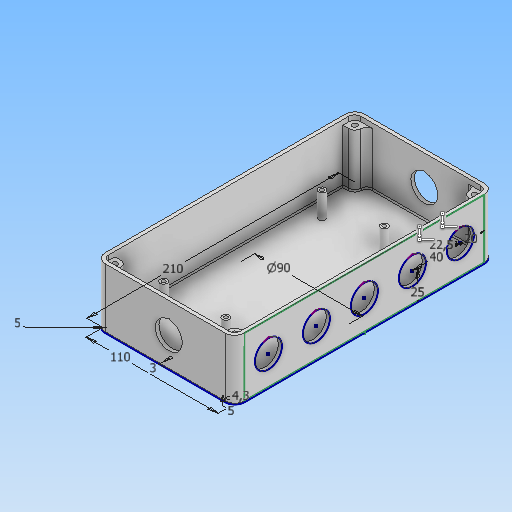
# Autodesk Inventor part: SchrackMulticlock_Box
Saved by Autodesk Inventor 2025.2 (Build 292293000, 293)
## iProperties
Created: 2024-12-26
Part Number: SchrackMulticlock_Box
Material: Všeobecné
Document SubType Name: Modeling
Designer: 42060
Density: 1 g/cm^3
Appearance: Výchozí
Author: 42060
Autodesk Inventor part; units mm, degrees
(part 1 of 2)
ref_plane "YZ Plane" through (0, 0, 0) normal (1, 0, 0) x (0, 1, 0)
ref_plane "XZ Plane" through (0, 0, 0) normal (0, 1, 0) x (-1, 0, 0)
ref_plane "XY Plane" through (0, 0, 0) normal (0, 0, 1) x (1, 0, 0)
sketch "PCB" plane through (0, 0, 0) normal (0, 1, 0) x (-1, 0, 0)
  line L0 (45, 45) -> (79, 45)
  line L1 (79, 45) -> (83.2426, 49.2426)
  line L2 (83.2426, 49.2426) -> (86.7426, 49.2426)
  line L3 (86.7426, 49.2426) -> (89.2426, 46.7426)
  line L4 (89.2426, 46.7426) -> (89.2426, 43.2426)
  line L5 (89.2426, 43.2426) -> (85, 39)
  line L6 (85, 39) -> (85, 0)
  circle A0 centre (85, 45) radius 1.6
  line L7 (85, 0) -> (45, 0)
  line L8 (45, 0) -> (45, 45)
  line L9 (45, -45) -> (79, -45)
  line L10 (79, -45) -> (83.2426, -49.2426)
  line L11 (83.2426, -49.2426) -> (86.7426, -49.2426)
  line L12 (86.7426, -49.2426) -> (89.2426, -46.7426)
  line L13 (89.2426, -46.7426) -> (89.2426, -43.2426)
  line L14 (89.2426, -43.2426) -> (85, -39)
  line L15 (85, -39) -> (85, 0)
  circle A1 centre (85, -45) radius 1.6
  line L16 (45, 45) -> (11, 45)
  line L17 (11, 45) -> (6.7574, 49.2426)
  line L18 (6.7574, 49.2426) -> (3.2574, 49.2426)
  line L19 (3.2574, 49.2426) -> (0.7574, 46.7426)
  line L20 (0.7574, 46.7426) -> (0.7574, 43.2426)
  line L21 (0.7574, 43.2426) -> (5, 39)
  line L22 (5, 39) -> (5, 0)
  circle A2 centre (5, 45) radius 1.6
  line L23 (45, -45) -> (11, -45)
  line L24 (11, -45) -> (6.7574, -49.2426)
  line L25 (6.7574, -49.2426) -> (3.2574, -49.2426)
  line L26 (3.2574, -49.2426) -> (0.7574, -46.7426)
  line L27 (0.7574, -46.7426) -> (0.7574, -43.2426)
  line L28 (0.7574, -43.2426) -> (5, -39)
  line L29 (5, -39) -> (5, 0)
  circle A3 centre (5, -45) radius 1.6
  line L30 (103.1723, 66.0113) -> (103.1723, -78.0847) construction
  line L31 (103.1723, -78.0847) -> (-10.5, -78.0847) construction
  line L32 (-10.5, -78.0847) -> (-10.5, 66.0113) construction
  line L33 (-10.5, 66.0113) -> (103.1723, 66.0113) construction
  line L34 (5, 40) -> (-75, 40)
  line L35 (-75, 40) -> (-75, -40)
  line L36 (-75, -40) -> (5, -40)
  line L37 (5, -40) -> (5, 40)
  line L38 (5, 40) -> (-75, -40) construction
  line L39 (-75, 40) -> (5, -40) construction
  circle A4 centre (-66, 31) radius 2
  line L40 (5, 0) -> (-75, 0)
  line L41 (-35, -40) -> (-35, 40)
  circle A5 centre (-66, -31) radius 2
  circle A6 centre (-4, 31) radius 2
  circle A7 centre (-4, -31) radius 2
  line L42 (-67.5, -40) -> (-67.5, 40) construction
  line L43 (-45, 55) -> (-90, 55)
  line L44 (-90, 55) -> (-90, 25)
  line L45 (-90, 25) -> (-45, 25)
  line L46 (-45, 25) -> (-45, 55)
  line L47 (-45, 55) -> (-90, 25) construction
  line L48 (-90, 55) -> (-45, 25) construction
  line L49 (-45, -15) -> (-45, 15)
  line L50 (-90, -15) -> (-45, -15)
  line L51 (-90, 15) -> (-90, -15)
  line L52 (-45, 15) -> (-90, 15)
  line L53 (-45, -55) -> (-45, -25)
  line L54 (-90, -55) -> (-45, -55)
  line L55 (-90, -25) -> (-90, -55)
  line L56 (-45, -25) -> (-90, -25)
  line L57 (76, 60.25) -> (14, 60.25)
  line L58 (14, 60.25) -> (14, 49.75)
  line L59 (14, 49.75) -> (76, 49.75)
  line L60 (76, 49.75) -> (76, 60.25)
  line L61 (76, 60.25) -> (14, 49.75) construction
  line L62 (14, 60.25) -> (76, 49.75) construction
  line L63 (-13.5, 26.75) -> (-56.5, 26.75)
  line L64 (-56.5, 26.75) -> (-56.5, -26.75)
  line L65 (-56.5, -26.75) -> (-13.5, -26.75)
  line L66 (-13.5, -26.75) -> (-13.5, 26.75)
  line L67 (-13.5, 26.75) -> (-56.5, -26.75) construction
  line L68 (-56.5, 26.75) -> (-13.5, -26.75) construction
  line L69 (-9, 26.75) -> (-61, 26.75)
  line L70 (-61, 26.75) -> (-61, -26.75)
  line L71 (-61, -26.75) -> (-9, -26.75)
  line L72 (-9, -26.75) -> (-9, 26.75)
  line L73 (-9, 26.75) -> (-61, -26.75) construction
  line L74 (-61, 26.75) -> (-9, -26.75) construction
  point P0 (0, 0)
  point P1 (0, 0)
  point P2 (-35, 0)
  point P3 (-67.5, 0)
  point P4 (45, 55)
  dimension "d2" = 6
  dimension "d3" = 39
  dimension "d4" = 34
  dimension "d5" = 40
  dimension "d6" = 45
  dimension "d7" = 3.5
  dimension "d8" = 3.2
  dimension "d11" = 45
  dimension "d65" = 80
  dimension "d66" = 80
  dimension "d68" = 80
  dimension "d69" = 4
  dimension "d70" = 31
  dimension "d83" = 55.5
  dimension "d87" = 144.096
  dimension "d91" = 66.0113
  dimension "d105" = 30
  dimension "d106" = 45
  dimension "d107" = 40
  dimension "d110" = 40
  dimension "d116" = 135
  dimension "d117" = 62
  dimension "d118" = 10.5
  dimension "d120" = 55
  dimension "d162" = 43
  dimension "d163" = 53.5
  dimension "d164" = 52
  constraints: 142 end point, 26 symmetric about line, 15 midpoint, 12 parallel, 9 horizontal, 9 perpendicular, 8 centre point, 5 horizontal alignment, 3 equal length, 3 vertical alignment, 2 vertical, 1 coincident, 1 point on line, 26 other
  measures "d2" distance of L4.end L5.end
  measures "d3" distance of L5.end L6.end
  measures "d4" distance of L0.start L0.end
  measures "d5" distance from line of L7.end L6
  measures "d6" distance from line of L7.end L0
  measures "d7" distance of L3.end L4.end
  measures "d8" diameter of A0
  measures "d11" distance of point (0, 0) L7.end
  measures "d65" distance of L35.end L36.end
  measures "d66" distance of L34.end L35.end
  measures "d68" distance of point (-35, 0) L7.end
  measures "d69" diameter of A4
  measures "d70" vertical distance of L40.end A4.centre
  measures "d83" distance from line of L7.end L32
  measures "d87" distance between parallel lines of L31 L33
  measures "d91" distance from line of L33 L7.end
  measures "d105" distance of L45.end L43.start
  measures "d106" distance of L44.end L45.end
  measures "d107" distance of L42.end point (-67.5, 0)
  measures "d110" distance of L45.end L49.start
  measures "d116" distance from line of L7.end L51
  measures "d117" distance of L58.end L59.end
  measures "d118" distance of L57.end L58.end
  measures "d120" distance of L7.end point (45, 55)
  measures "d162" distance of L63.start L63.end
  measures "d163" distance of L65.end L63.start
  measures "d164" distance of L70.end L71.end
sketch "Náčrt2" plane through (0, 0, 0) normal (0, 1, 0) x (-1, 0, 0)
  line L0 (50, 105) -> (-40, 105)
  line L1 (-55, 90) -> (-55, -100)
  line L2 (-50, -105) -> (50, -105)
  line L3 (55, -100) -> (55, 100)
  line L4 (55, 105) -> (-55, -105) construction
  line L5 (-55, 105) -> (55, -105) construction
  arc A0 (55, 100) -> (50, 105) centre (50, 100) ccw
  arc A1 (50, -105) -> (55, -100) centre (50, -100) ccw
  arc A2 (-55, -100) -> (-50, -105) centre (-50, -100) ccw
  arc A3 (-50, 105) -> (-55, 100) centre (-50, 100) ccw
  line L6 (-50, 108) -> (50, 108)
  arc A4 (58, 100) -> (50, 108) centre (50, 100) ccw
  line L7 (58, 100) -> (58, -100)
  arc A5 (50, -108) -> (58, -100) centre (50, -100) ccw
  line L8 (50, -108) -> (-50, -108)
  arc A6 (-58, -100) -> (-50, -108) centre (-50, -100) ccw
  line L9 (-58, -100) -> (-58, 100)
  arc A7 (-50, 108) -> (-58, 100) centre (-50, 100) ccw
  circle A8 centre (-50, 100) radius 5
  line L10 (-45, 100) -> (-45, 100)
  line L11 (-50, 95) -> (-50, 95)
  arc A9 (-40, 105) -> (-45, 100) centre (-40, 100) ccw
  arc A10 (-50, 95) -> (-55, 90) centre (-50, 90) ccw
  line L12 (-40, 105) -> (-50, 105)
  line L13 (-55, 90) -> (-55, 100)
  circle A11 centre (-50, 100) radius 2.15
  line L14 (55, 0) -> (-55, 0)
  line L15 (0, 105) -> (0, -105)
  circle A12 centre (-50, -100) radius 5
  arc A13 (-45, -100) -> (-40, -105) centre (-40, -100) ccw
  arc A14 (-55, -90) -> (-50, -95) centre (-50, -90) ccw
  circle A15 centre (-50, -100) radius 2.15
  circle A16 centre (50, 100) radius 5
  line L16 (45, 100) -> (45, 100)
  line L17 (50, 95) -> (50, 95)
  arc A17 (45, 100) -> (40, 105) centre (40, 100) ccw
  arc A18 (55, 90) -> (50, 95) centre (50, 90) ccw
  circle A19 centre (50, 100) radius 2.15
  arc A20 (50, -95) -> (55, -90) centre (50, -90) ccw
  circle A21 centre (50, -100) radius 2.15
  arc A22 (40, -105) -> (45, -100) centre (40, -100) ccw
  circle A23 centre (50, -100) radius 5
  line L18 (-50, 95) -> (-55, 95)
  line L19 (-50, -95) -> (-55, -95)
  line L20 (50, 95) -> (55, 95)
  line L21 (50, -95) -> (55, -95)
  point P0 (0, 0)
  point P1 (-45, 100)
  point P2 (-55, 100)
  point P3 (-45, -100)
  point P4 (-50, -95)
  point P5 (50, -100)
  point P6 (45, -100)
  point P7 (50, -95)
  point P8 (-40, -105)
  point P9 (-45, -100)
  point P10 (-50, -95)
  point P11 (50, -95)
  point P12 (40, -105)
  point P13 (45, 100)
  point P14 (40, 105)
  point P15 (55, 95)
  point P16 (50, -95)
  point P17 (-50, -95)
  point P18 (45, 0)
  point P19 (0, 0)
  dimension "d9" = 210
  dimension "d10" = 110
  dimension "d12" = 5
  dimension "d124" = 3
  dimension "d136" = 5
  dimension "d137" = 4.3
  dimension "d525" = 90
  constraints: 44 end point, 41 point on circle, 40 symmetric about line, 24 centre point, 16 tangent, 13 point on line, 8 coincident, 6 midpoint, 5 equal radius, 4 parallel, 4 perpendicular, 3 horizontal, 2 vertical, 1 horizontal alignment, 19 other
  measures "d9" distance of L5.end L4.start
  measures "d10" distance of L4.start L5.start
  measures "d12" radius of A0
  measures "d124" distance between parallel lines of L0 L6
  measures "d136" radius of A9
  measures "d137" diameter of A11
  measures "d525" diameter of point (45, 0) point (0, 0)
extrude "Vysunutí1" add sketch "Náčrt2" along normal blind 2 contours A16 A17 L0 | A0 A16 | A17 A16 A18 L3 L14 L15 L0 | L3 L20 A16 | L15 L14 L1 A10 A8 A9 L0 | L3 A18 L20 | A9 A8 L12 | L15 L2 A13 A12 A14 L1 L14 | L14 L3 A20 A23 A22 L2 L15 | A8 A3 | L18 L13 A8 | A10 L13 L18 | L3 L21 A20 | A14 L19 L1 | L2 A12 A13 | A22 A23 L2 | L3 A23 L21 | A23 A1 | L19 A12 L1 | A12 A2 | L6 A4 L7 A5 L8 A6 L9 A7 | A11 | A15 | A19 | A21
extrude "Vysunutí2" add sketch "Náčrt2" along normal blind 50 contours L6 A4 L7 A5 L8 A6 L9 A7
extrude "Vysunutí4" add sketch "Náčrt2" along normal blind 46 contours A16 A17 L0 | A0 A16 | L3 L20 A16 | A9 A8 L12 | A8 A3 | L18 L13 A8 | L2 A12 A13 | A22 A23 L2 | L3 A23 L21 | A23 A1 | L19 A12 L1 | A12 A2
chamfer "Zkosení1" distance 1 angle 45 8 edges at (58, 0, 0) (55.6569, 0, -105.6569) (0, 0, -108) (-55.6569, 0, -105.6569) (-58, 0, 0) (-55.6569, 0, 105.6569) (0, 0, 108) (55.6569, 0, 105.6569)
chamfer "Zkosení2" distance 1 angle 45 16 edges at (-46.4645, 2, 96.4645) (-43.5355, 2, 103.5355) (0, 2, 105) (43.5355, 2, 103.5355) (46.4645, 2, 96.4645) (52.5, 2, 95) (-52.5, 2, 95) (-55, 2, 0) (0, 2, -105) (-43.5355, 2, -103.5355) (-46.4645, 2, -96.4645) (-52.5, 2, -95) (43.5355, 2, -103.5355) (46.4645, 2, -96.4645) (52.5, 2, -95) (55, 2, 0)
ref_plane "Pracovní rovina1" through (0, 36, 0) normal (0, 1, 0) x (1, 0, 0)
sketch "Náčrt6" plane through (58, 50, 100) normal (1, 0, 0) x (0, 0, -1)
  circle A0 centre (180, -25) radius 11.25
  line L0 (176.0852, -14.4531) -> (180, -13)
  line L1 (180, -13) -> (183.9148, -14.4531)
  line L2 (0, -50) -> (200, -50) projected
  line L3 (200, -49) -> (200, 0) projected
  line L4 (200, -49) -> (0, -49) projected
  line L5 (200, -49) -> (200, 0) projected
  line L6 (0, 0) -> (200, 0) projected
  line L7 (0, -49) -> (0, 0) projected
  circle A1 centre (140, -25) radius 11.25
  line L8 (136.0852, -14.4531) -> (140, -13)
  line L9 (140, -13) -> (143.9148, -14.4531)
  circle A2 centre (100, -25) radius 11.25
  line L10 (96.0852, -14.4531) -> (100, -13)
  line L11 (100, -13) -> (103.9148, -14.4531)
  circle A3 centre (60, -25) radius 11.25
  line L12 (56.0852, -14.4531) -> (60, -13)
  line L13 (60, -13) -> (63.9148, -14.4531)
  circle A4 centre (20, -25) radius 11.25
  line L14 (16.0852, -14.4531) -> (20, -13)
  line L15 (20, -13) -> (23.9148, -14.4531)
  point P0 (100, -50)
  point P1 (182.4515, -14.0204)
  dimension "d609" = 22.5
  dimension "d610" = 25
  dimension "d611" = 20
  dimension "d614" = 40
  constraints: 20 end point, 10 point on circle, 5 centre point, 2 tangent, 1 horizontal, 28 other
  measures "d609" diameter of A0
  measures "d610" distance from line of L2 A0.centre
  measures "d611" distance from line of L3 A0.centre
  measures "d614" distance of A0.centre A1.centre
extrude "Vysunutí8" cut sketch "Náčrt6" against normal up to surface (3 mm away) contours A0 | A0 L0 L1 | A1 | A1 L8 L9 | A2 | A2 L10 L11 | A3 | A3 L12 L13 | A4 | A4 L14 L15
sketch "Sketch16" plane through (-58, 50, -100) normal (-1, 0, 0) x (0, 0, 1)
  line L0 (83.6122, -35.7493) -> (81.9759, -35.7493)
  line L1 (81.9759, -35.7493) -> (81.7423, -35.786)
  line L2 (81.7423, -35.786) -> (81.5927, -35.8771)
  line L3 (81.5927, -35.8771) -> (81.4287, -36.1113)
  line L4 (81.4287, -36.1113) -> (81.2378, -36.3119)
  line L5 (81.2378, -36.3119) -> (81.0126, -36.3763)
  line L6 (81.0126, -36.3763) -> (80.8497, -36.3769)
  line L7 (80.8497, -36.3769) -> (80.6856, -36.3485)
  line L8 (80.6856, -36.3485) -> (80.6027, -36.2609)
  line L9 (80.6027, -36.2609) -> (80.6707, -35.9053)
  line L10 (80.6707, -35.9053) -> (81.9875, -33.1293)
  line L11 (81.9875, -33.1293) -> (82.2034, -32.8403)
  line L12 (82.2034, -32.8403) -> (82.5118, -32.7443)
  line L13 (82.5118, -32.7443) -> (82.8391, -32.7481)
  line L14 (82.8391, -32.7481) -> (83.0353, -32.858)
  line L15 (83.0353, -32.858) -> (83.0612, -33.0921)
  line L16 (83.0612, -33.0921) -> (83.0433, -33.383)
  line L17 (83.0433, -33.383) -> (83.12, -33.4728)
  line L18 (83.12, -33.4728) -> (83.2556, -33.506)
  line L19 (83.2556, -33.506) -> (84.7242, -33.506)
  line L20 (84.7242, -33.506) -> (84.9963, -33.4315)
  line L21 (84.9963, -33.4315) -> (85.2006, -33.235)
  line L22 (85.2006, -33.235) -> (85.3303, -32.9572)
  line L23 (85.3303, -32.9572) -> (85.3787, -32.6387)
  line L24 (85.3787, -32.6387) -> (85.3391, -32.3203)
  line L25 (85.3391, -32.3203) -> (85.2049, -32.0425)
  line L26 (85.2049, -32.0425) -> (84.9692, -31.846)
  line L27 (84.9692, -31.846) -> (84.6255, -31.7714)
  line L28 (84.6255, -31.7714) -> (81.2636, -31.7714)
  line L29 (81.2636, -31.7714) -> (80.806, -31.8484)
  line L30 (80.806, -31.8484) -> (80.4005, -32.0677)
  line L31 (80.4005, -32.0677) -> (80.0566, -32.4122)
  line L32 (80.0566, -32.4122) -> (79.7838, -32.8649)
  line L33 (79.7838, -32.8649) -> (78.2065, -36.2017)
  line L34 (78.2065, -36.2017) -> (78.0796, -36.6902)
  line L35 (78.0796, -36.6902) -> (78.1692, -37.0583)
  line L36 (78.1692, -37.0583) -> (78.4033, -37.2907)
  line L37 (78.4033, -37.2907) -> (78.7097, -37.3716)
  line L38 (78.7097, -37.3716) -> (82.3161, -37.3716)
  line L39 (82.3161, -37.3716) -> (82.7872, -37.3019)
  line L40 (82.7872, -37.3019) -> (83.1788, -37.1181)
  line L41 (83.1788, -37.1181) -> (83.4864, -36.8583)
  line L42 (83.4864, -36.8583) -> (83.7057, -36.5605)
  line L43 (83.7057, -36.5605) -> (83.8322, -36.2626)
  line L44 (83.8322, -36.2626) -> (83.8618, -36.0028)
  line L45 (83.8618, -36.0028) -> (83.7899, -35.819)
  line L46 (83.7899, -35.819) -> (83.6122, -35.7493)
  line L47 (72.2106, -32.761) -> (72.4074, -32.7104)
  line L48 (72.4074, -32.7104) -> (72.5473, -32.5627)
  line L49 (72.5473, -32.5627) -> (72.5797, -32.4966)
  line L50 (72.5797, -32.4966) -> (72.6457, -32.3535)
  line L51 (72.6457, -32.3535) -> (72.6482, -32.349)
  line L52 (72.6482, -32.349) -> (72.7793, -32.0641)
  line L53 (72.7793, -32.0641) -> (72.7841, -31.8728)
  line L54 (72.7841, -31.8728) -> (72.7229, -31.8003)
  line L55 (72.7229, -31.8003) -> (72.609, -31.7714)
  line L56 (72.609, -31.7714) -> (70.745, -31.7657)
  line L57 (70.745, -31.7657) -> (70.7334, -31.7689)
  line L58 (70.7334, -31.7689) -> (67.6082, -31.7689)
  line L59 (67.6082, -31.7689) -> (66.5311, -31.7657)
  line L60 (66.5311, -31.7657) -> (66.4384, -31.7817)
  line L61 (66.4384, -31.7817) -> (66.3006, -31.8437)
  line L62 (66.3006, -31.8437) -> (66.1974, -31.9653)
  line L63 (66.1974, -31.9653) -> (66.1651, -32.0223)
  line L64 (66.1651, -32.0223) -> (66.0672, -32.2303)
  line L65 (66.0672, -32.2303) -> (66.0728, -32.2303)
  line L66 (66.0728, -32.2303) -> (65.9641, -32.4671)
  line L67 (65.9641, -32.4671) -> (65.9591, -32.6573)
  line L68 (65.9591, -32.6573) -> (66.0197, -32.73)
  line L69 (66.0197, -32.73) -> (66.1332, -32.759)
  line L70 (66.1332, -32.759) -> (66.5122, -32.7603)
  line L71 (66.5122, -32.7603) -> (66.5122, -32.761)
  line L72 (66.5122, -32.761) -> (67.4629, -32.761)
  line L73 (67.4629, -32.761) -> (67.9984, -32.7635)
  line L74 (67.9984, -32.7635) -> (67.9997, -32.761)
  line L75 (67.9997, -32.761) -> (68.0321, -32.761)
  line L76 (68.0321, -32.761) -> (66.0465, -37.0661)
  line L77 (66.0465, -37.0661) -> (66.0469, -37.2892)
  line L78 (66.0469, -37.2892) -> (66.2073, -37.3915)
  line L79 (66.2073, -37.3915) -> (66.4833, -37.3915)
  line L80 (66.4833, -37.3915) -> (67.8656, -37.3915)
  line L81 (67.8656, -37.3915) -> (67.9721, -37.3895)
  line L82 (67.9721, -37.3895) -> (68.1683, -37.3379)
  line L83 (68.1683, -37.3379) -> (68.3102, -37.19)
  line L84 (68.3102, -37.19) -> (68.5042, -36.7838)
  line L85 (68.5042, -36.7838) -> (68.5046, -36.7838)
  line L86 (68.5046, -36.7838) -> (68.5637, -36.6586)
  line L87 (68.5637, -36.6586) -> (68.5663, -36.6529)
  line L88 (68.5663, -36.6529) -> (68.8155, -36.1164)
  line L89 (68.8155, -36.1164) -> (68.856, -36.0285)
  line L90 (68.856, -36.0285) -> (68.9104, -35.9123)
  line L91 (68.9104, -35.9123) -> (69.9435, -33.6927)
  line L92 (69.9435, -33.6927) -> (70.3078, -32.9111)
  line L93 (70.3078, -32.9111) -> (70.398, -32.8193)
  line L94 (70.398, -32.8193) -> (70.5648, -32.7635)
  line L95 (70.5648, -32.7635) -> (70.8183, -32.7635)
  line L96 (70.8183, -32.7635) -> (70.8183, -32.761)
  line L97 (70.8183, -32.761) -> (71.9394, -32.761)
  line L98 (71.9394, -32.761) -> (72.2106, -32.761)
  line L99 (77.0928, -36.3955) -> (75.2413, -36.3955)
  line L100 (75.2413, -36.3955) -> (73.931, -36.3955)
  line L101 (73.931, -36.3955) -> (73.8331, -36.3352)
  line L102 (73.8331, -36.3352) -> (73.8323, -36.1979)
  line L103 (73.8323, -36.1979) -> (73.8693, -36.1164)
  line L104 (73.8693, -36.1164) -> (74.279, -35.2373)
  line L105 (74.279, -35.2373) -> (74.3685, -35.1443)
  line L106 (74.3685, -35.1443) -> (74.5372, -35.0884)
  line L107 (74.5372, -35.0884) -> (75.165, -35.0865)
  line L108 (75.165, -35.0865) -> (76.1951, -35.0865)
  line L109 (76.1951, -35.0865) -> (76.4663, -35.0865)
  line L110 (76.4663, -35.0865) -> (76.6641, -35.0349)
  line L111 (76.6641, -35.0349) -> (76.8056, -34.8875)
  line L112 (76.8056, -34.8875) -> (76.8341, -34.8214)
  line L113 (76.8341, -34.8214) -> (76.9022, -34.679)
  line L114 (76.9022, -34.679) -> (76.9048, -34.6726)
  line L115 (76.9048, -34.6726) -> (77.0773, -34.3228)
  line L116 (77.0773, -34.3228) -> (77.0823, -34.1311)
  line L117 (77.0823, -34.1311) -> (77.0216, -34.0581)
  line L118 (77.0216, -34.0581) -> (76.9091, -34.029)
  line L119 (76.9091, -34.029) -> (76.6871, -34.029)
  line L120 (76.6871, -34.029) -> (76.6897, -34.0264)
  line L121 (76.6897, -34.0264) -> (75.0378, -34.0264)
  line L122 (75.0378, -34.0264) -> (74.9399, -33.966)
  line L123 (74.9399, -33.966) -> (74.9387, -33.8281)
  line L124 (74.9387, -33.8281) -> (75.0469, -33.5913)
  line L125 (75.0469, -33.5913) -> (75.0413, -33.5939)
  line L126 (75.0413, -33.5939) -> (75.3621, -32.9124)
  line L127 (75.3621, -32.9124) -> (75.4507, -32.8201)
  line L128 (75.4507, -32.8201) -> (75.6173, -32.7648)
  line L129 (75.6173, -32.7648) -> (75.8696, -32.7635)
  line L130 (75.8696, -32.7635) -> (75.8696, -32.761)
  line L131 (75.8696, -32.761) -> (76.4163, -32.761)
  line L132 (76.4163, -32.761) -> (76.4529, -32.761)
  line L133 (76.4529, -32.761) -> (78.5752, -32.761)
  line L134 (78.5752, -32.761) -> (78.849, -32.761)
  line L135 (78.849, -32.761) -> (79.0453, -32.7104)
  line L136 (79.0453, -32.7104) -> (79.1853, -32.5627)
  line L137 (79.1853, -32.5627) -> (79.2159, -32.4966)
  line L138 (79.2159, -32.4966) -> (79.2823, -32.3535)
  line L139 (79.2823, -32.3535) -> (79.2849, -32.349)
  line L140 (79.2849, -32.349) -> (79.4164, -32.0641)
  line L141 (79.4164, -32.0641) -> (79.4213, -31.8728)
  line L142 (79.4213, -31.8728) -> (79.3604, -31.8003)
  line L143 (79.3604, -31.8003) -> (79.247, -31.7714)
  line L144 (79.247, -31.7714) -> (77.3821, -31.7657)
  line L145 (77.3821, -31.7657) -> (77.3701, -31.7689)
  line L146 (77.3701, -31.7689) -> (74.871, -31.7689)
  line L147 (74.871, -31.7689) -> (73.7952, -31.7657)
  line L148 (73.7952, -31.7657) -> (73.5825, -31.837)
  line L149 (73.5825, -31.837) -> (73.4274, -32.0223)
  line L150 (73.4274, -32.0223) -> (71.1012, -37.0674)
  line L151 (71.1012, -37.0674) -> (71.0998, -37.2903)
  line L152 (71.0998, -37.2903) -> (71.2607, -37.3934)
  line L153 (71.2607, -37.3934) -> (74.0004, -37.3934)
  line L154 (74.0004, -37.3934) -> (74.0004, -37.3915)
  line L155 (74.0004, -37.3915) -> (74.8481, -37.3915)
  line L156 (74.8481, -37.3915) -> (74.8494, -37.3934)
  line L157 (74.8494, -37.3934) -> (75.1323, -37.3915)
  line L158 (75.1323, -37.3915) -> (76.2335, -37.3902)
  line L159 (76.2335, -37.3902) -> (76.6871, -37.387)
  line L160 (76.6871, -37.387) -> (76.8834, -37.3347)
  line L161 (76.8834, -37.3347) -> (77.0251, -37.1868)
  line L162 (77.0251, -37.1868) -> (77.1273, -36.9724)
  line L163 (77.1273, -36.9724) -> (77.1299, -36.9724)
  line L164 (77.1299, -36.9724) -> (77.2614, -36.6869)
  line L165 (77.2614, -36.6869) -> (77.2667, -36.4962)
  line L166 (77.2667, -36.4962) -> (77.206, -36.4242)
  line L167 (77.206, -36.4242) -> (77.0928, -36.3955)
  line L168 (101.0813, -31.7529) -> (99.2173, -31.749)
  line L169 (99.2173, -31.749) -> (99.0057, -31.8191)
  line L170 (99.0057, -31.8191) -> (98.85, -32.0038)
  line L171 (98.85, -32.0038) -> (98.2226, -33.3763)
  line L172 (98.2226, -33.3763) -> (96.9718, -31.9492)
  line L173 (96.9718, -31.9492) -> (96.6999, -31.7788)
  line L174 (96.6999, -31.7788) -> (96.4358, -31.749)
  line L175 (96.4358, -31.749) -> (95.0448, -31.749)
  line L176 (95.0448, -31.749) -> (95.044, -31.749)
  line L177 (95.044, -31.749) -> (95.003, -31.749)
  line L178 (95.003, -31.749) -> (94.792, -31.8191)
  line L179 (94.792, -31.8191) -> (94.6365, -32.0038)
  line L180 (94.6365, -32.0038) -> (92.3086, -37.0494)
  line L181 (92.3086, -37.0494) -> (92.3086, -37.2719)
  line L182 (92.3086, -37.2719) -> (92.4703, -37.3741)
  line L183 (92.4703, -37.3741) -> (94.2325, -37.3683)
  line L184 (94.2325, -37.3683) -> (94.4295, -37.3165)
  line L185 (94.4295, -37.3165) -> (94.5706, -37.1688)
  line L186 (94.5706, -37.1688) -> (95.1013, -36.0477)
  line L187 (95.1013, -36.0477) -> (96.2853, -33.5072)
  line L188 (96.2853, -33.5072) -> (97.5263, -34.885)
  line L189 (97.5263, -34.885) -> (96.9886, -36.0503)
  line L190 (96.9886, -36.0503) -> (96.5221, -37.0494)
  line L191 (96.5221, -37.0494) -> (96.5221, -37.2719)
  line L192 (96.5221, -37.2719) -> (96.6825, -37.3741)
  line L193 (96.6825, -37.3741) -> (98.5223, -37.3683)
  line L194 (98.5223, -37.3683) -> (98.7179, -37.3165)
  line L195 (98.7179, -37.3165) -> (98.8586, -37.1688)
  line L196 (98.8586, -37.1688) -> (101.2508, -32.0455)
  line L197 (101.2508, -32.0455) -> (101.2559, -31.8544)
  line L198 (101.2559, -31.8544) -> (101.1949, -31.7818)
  line L199 (101.1949, -31.7818) -> (101.0813, -31.7529)
  line L200 (104.1263, -33.8242) -> (104.9718, -31.9973)
  line L201 (104.9718, -31.9973) -> (104.9627, -31.8423)
  line L202 (104.9627, -31.8423) -> (104.8287, -31.7503)
  line L203 (104.8287, -31.7503) -> (102.9901, -31.7464)
  line L204 (102.9901, -31.7464) -> (102.7787, -31.8168)
  line L205 (102.7787, -31.8168) -> (102.6245, -32.0012)
  line L206 (102.6245, -32.0012) -> (100.2957, -37.0462)
  line L207 (100.2957, -37.0462) -> (100.296, -37.2695)
  line L208 (100.296, -37.2695) -> (100.4583, -37.3716)
  line L209 (100.4583, -37.3716) -> (102.2209, -37.3664)
  line L210 (102.2209, -37.3664) -> (102.4162, -37.3142)
  line L211 (102.4162, -37.3142) -> (102.5572, -37.1662)
  line L212 (102.5572, -37.1662) -> (102.9375, -36.3692)
  line L213 (102.9375, -36.3692) -> (102.9358, -36.3673)
  line L214 (102.9358, -36.3673) -> (104.1263, -33.8242)
  line L215 (112.3462, -32.0089) -> (112.3875, -31.8192)
  line L216 (112.3875, -31.8192) -> (112.2445, -31.7464)
  line L217 (112.2445, -31.7464) -> (110.8526, -31.749)
  line L218 (110.8526, -31.749) -> (110.5884, -31.7788)
  line L219 (110.5884, -31.7788) -> (110.3167, -31.9492)
  line L220 (110.3167, -31.9492) -> (108.4738, -34.0328)
  line L221 (108.4738, -34.0328) -> (108.2728, -34.1494)
  line L222 (108.2728, -34.1494) -> (108.0164, -34.1888)
  line L223 (108.0164, -34.1888) -> (107.6313, -34.1778)
  line L224 (107.6313, -34.1778) -> (107.7529, -33.8981)
  line L225 (107.7529, -33.8981) -> (108.6317, -31.998)
  line L226 (108.6317, -31.998) -> (108.6227, -31.8451)
  line L227 (108.6227, -31.8451) -> (108.4885, -31.7509)
  line L228 (108.4885, -31.7509) -> (106.659, -31.749)
  line L229 (106.659, -31.749) -> (106.4504, -31.8187)
  line L230 (106.4504, -31.8187) -> (106.2955, -32.0025)
  line L231 (106.2955, -32.0025) -> (103.9805, -37.0225)
  line L232 (103.9805, -37.0225) -> (103.9801, -37.2443)
  line L233 (103.9801, -37.2443) -> (104.1401, -37.3453)
  line L234 (104.1401, -37.3453) -> (105.8928, -37.3408)
  line L235 (105.8928, -37.3408) -> (106.0892, -37.2885)
  line L236 (106.0892, -37.2885) -> (106.2296, -37.1418)
  line L237 (106.2296, -37.1418) -> (107.0544, -35.3868)
  line L238 (107.0544, -35.3868) -> (107.1171, -35.2953)
  line L239 (107.1171, -35.2953) -> (107.2575, -35.2398)
  line L240 (107.2575, -35.2398) -> (107.7818, -35.2398)
  line L241 (107.7818, -35.2398) -> (107.8923, -35.2894)
  line L242 (107.8923, -35.2894) -> (107.9495, -35.4246)
  line L243 (107.9495, -35.4246) -> (108.3885, -37.0225)
  line L244 (108.3885, -37.0225) -> (108.4801, -37.2488)
  line L245 (108.4801, -37.2488) -> (108.6394, -37.3453)
  line L246 (108.6394, -37.3453) -> (110.456, -37.3408)
  line L247 (110.456, -37.3408) -> (110.6422, -37.2264)
  line L248 (110.6422, -37.2264) -> (110.6754, -36.982)
  line L249 (110.6754, -36.982) -> (110.083, -35.0326)
  line L250 (110.083, -35.0326) -> (110.0374, -34.8084)
  line L251 (110.0374, -34.8084) -> (110.0393, -34.6576)
  line L252 (110.0393, -34.6576) -> (110.0912, -34.5327)
  line L253 (110.0912, -34.5327) -> (112.3462, -32.0089)
  line L254 (93.1153, -31.7503) -> (91.2496, -31.7464)
  line L255 (91.2496, -31.7464) -> (91.0384, -31.8168)
  line L256 (91.0384, -31.8168) -> (90.8827, -32.0012)
  line L257 (90.8827, -32.0012) -> (89.9889, -33.9532)
  line L258 (89.9889, -33.9532) -> (89.8987, -34.0564)
  line L259 (89.8987, -34.0564) -> (89.7591, -34.1047)
  line L260 (89.7591, -34.1047) -> (88.2344, -34.1047)
  line L261 (88.2344, -34.1047) -> (88.1365, -34.0441)
  line L262 (88.1365, -34.0441) -> (88.1339, -33.907)
  line L263 (88.1339, -33.907) -> (89.0166, -31.9973)
  line L264 (89.0166, -31.9973) -> (89.0093, -31.8423)
  line L265 (89.0093, -31.8423) -> (88.8756, -31.7503)
  line L266 (88.8756, -31.7503) -> (87.0366, -31.7464)
  line L267 (87.0366, -31.7464) -> (86.8251, -31.8168)
  line L268 (86.8251, -31.8168) -> (86.6701, -32.0012)
  line L269 (86.6701, -32.0012) -> (84.3418, -37.0462)
  line L270 (84.3418, -37.0462) -> (84.3425, -37.2695)
  line L271 (84.3425, -37.2695) -> (84.5043, -37.3716)
  line L272 (84.5043, -37.3716) -> (86.2665, -37.3664)
  line L273 (86.2665, -37.3664) -> (86.4627, -37.3142)
  line L274 (86.4627, -37.3142) -> (86.6028, -37.1662)
  line L275 (86.6028, -37.1662) -> (87.4755, -35.3156)
  line L276 (87.4755, -35.3156) -> (87.5654, -35.2235)
  line L277 (87.5654, -35.2235) -> (87.7325, -35.168)
  line L278 (87.7325, -35.168) -> (89.2046, -35.168)
  line L279 (89.2046, -35.168) -> (89.3275, -35.2218)
  line L280 (89.3275, -35.2218) -> (89.3382, -35.3541)
  line L281 (89.3382, -35.3541) -> (88.5561, -37.0462)
  line L282 (88.5561, -37.0462) -> (88.5553, -37.2695)
  line L283 (88.5553, -37.2695) -> (88.7165, -37.3716)
  line L284 (88.7165, -37.3716) -> (90.555, -37.3664)
  line L285 (90.555, -37.3664) -> (90.751, -37.3142)
  line L286 (90.751, -37.3142) -> (90.8918, -37.1662)
  line L287 (90.8918, -37.1662) -> (93.2839, -32.0429)
  line L288 (93.2839, -32.0429) -> (93.2897, -31.8518)
  line L289 (93.2897, -31.8518) -> (93.2287, -31.7792)
  line L290 (93.2287, -31.7792) -> (93.1153, -31.7503)
  line L291 (69.1316, -21.2213) -> (68.7219, -22.1875)
  line L292 (68.7219, -22.1875) -> (68.286, -23.0873)
  line L293 (68.286, -23.0873) -> (68.0867, -23.3387)
  line L294 (68.0867, -23.3387) -> (67.8128, -23.5656)
  line L295 (67.8128, -23.5656) -> (67.5032, -23.7299)
  line L296 (67.5032, -23.7299) -> (67.1969, -23.7932)
  line L297 (67.1969, -23.7932) -> (64.7042, -23.7932)
  line L298 (64.7042, -23.7932) -> (64.5512, -23.7017)
  line L299 (64.5512, -23.7017) -> (64.5443, -23.525)
  line L300 (64.5443, -23.525) -> (65.8378, -20.6977)
  line L301 (65.8378, -20.6977) -> (66.0185, -20.4497)
  line L302 (66.0185, -20.4497) -> (66.294, -20.3736)
  line L303 (66.294, -20.3736) -> (68.687, -20.3736)
  line L304 (68.687, -20.3736) -> (68.9816, -20.4465)
  line L305 (68.9816, -20.4465) -> (69.151, -20.6386)
  line L306 (69.151, -20.6386) -> (69.1996, -20.9102)
  line L307 (69.1996, -20.9102) -> (69.1316, -21.2213)
  line L308 (69.608, -25.4501) -> (70.3446, -25.2061)
  line L309 (70.3446, -25.2061) -> (71.3036, -24.7685)
  line L310 (71.3036, -24.7685) -> (71.796, -24.474)
  line L311 (71.796, -24.474) -> (72.2594, -24.1273)
  line L312 (72.2594, -24.1273) -> (72.6656, -23.7271)
  line L313 (72.6656, -23.7271) -> (72.9863, -23.2722)
  line L314 (72.9863, -23.2722) -> (73.4315, -22.4084)
  line L315 (73.4315, -22.4084) -> (73.878, -21.3195)
  line L316 (73.878, -21.3195) -> (74.0204, -20.7885)
  line L317 (74.0204, -20.7885) -> (74.0423, -20.2671)
  line L318 (74.0423, -20.2671) -> (73.9482, -19.774)
  line L319 (73.9482, -19.774) -> (73.7428, -19.3283)
  line L320 (73.7428, -19.3283) -> (73.4306, -18.9487)
  line L321 (73.4306, -18.9487) -> (73.0161, -18.6542)
  line L322 (73.0161, -18.6542) -> (72.504, -18.4636)
  line L323 (72.504, -18.4636) -> (71.8989, -18.3959)
  line L324 (71.8989, -18.3959) -> (62.6911, -18.3959)
  line L325 (62.6911, -18.3959) -> (62.2679, -18.4629)
  line L326 (62.2679, -18.4629) -> (62.057, -18.597)
  line L327 (62.057, -18.597) -> (61.8787, -18.8432)
  line L328 (61.8787, -18.8432) -> (56.9914, -29.3215)
  line L329 (56.9914, -29.3215) -> (56.9573, -29.4987)
  line L330 (56.9573, -29.4987) -> (57.015, -29.6296)
  line L331 (57.015, -29.6296) -> (57.2621, -29.7386)
  line L332 (57.2621, -29.7386) -> (61.0992, -29.7386)
  line L333 (61.0992, -29.7386) -> (61.5204, -29.6258)
  line L334 (61.5204, -29.6258) -> (61.6925, -29.4944)
  line L335 (61.6925, -29.4944) -> (61.8136, -29.3215)
  line L336 (61.8136, -29.3215) -> (63.4784, -25.7446)
  line L337 (63.4784, -25.7446) -> (63.6102, -25.6009)
  line L338 (63.6102, -25.6009) -> (63.7751, -25.5592)
  line L339 (63.7751, -25.5592) -> (64.9755, -25.5611)
  line L340 (64.9755, -25.5611) -> (64.994, -25.5611)
  line L341 (64.994, -25.5611) -> (65.1727, -25.6306)
  line L342 (65.1727, -25.6306) -> (65.2398, -25.7902)
  line L343 (65.2398, -25.7902) -> (65.1617, -29.3189)
  line L344 (65.1617, -29.3189) -> (65.1904, -29.4971)
  line L345 (65.1904, -29.4971) -> (65.2802, -29.6288)
  line L346 (65.2802, -29.6288) -> (65.5869, -29.7386)
  line L347 (65.5869, -29.7386) -> (69.5127, -29.7386)
  line L348 (69.5127, -29.7386) -> (69.8204, -29.6338)
  line L349 (69.8204, -29.6338) -> (69.9063, -29.5007)
  line L350 (69.9063, -29.5007) -> (69.9318, -29.3105)
  line L351 (69.9318, -29.3105) -> (69.6595, -27.7726)
  line L352 (69.6595, -27.7726) -> (69.3519, -25.8062)
  line L353 (69.3519, -25.8062) -> (69.4348, -25.5726)
  line L354 (69.4348, -25.5726) -> (69.608, -25.4501)
  line L355 (80.7772, -25.8903) -> (80.6946, -26.0892)
  line L356 (80.6946, -26.0892) -> (80.5159, -26.1611)
  line L357 (80.5159, -26.1611) -> (77.6094, -26.1611)
  line L358 (77.6094, -26.1611) -> (77.4327, -26.0894)
  line L359 (77.4327, -26.0894) -> (77.4087, -26.0046)
  line L360 (77.4087, -26.0046) -> (77.4584, -25.8916)
  line L361 (77.4584, -25.8916) -> (79.2696, -23.1976)
  line L362 (79.2696, -23.1976) -> (80.7367, -20.9646)
  line L363 (80.7367, -20.9646) -> (80.8715, -20.8291)
  line L364 (80.8715, -20.8291) -> (80.9666, -20.8133)
  line L365 (80.9666, -20.8133) -> (81.0351, -20.9781)
  line L366 (81.0351, -20.9781) -> (80.7772, -25.8903)
  line L367 (85.205, -18.3876) -> (79.986, -18.3876)
  line L368 (79.986, -18.3876) -> (79.6705, -18.4224)
  line L369 (79.6705, -18.4224) -> (79.3694, -18.524)
  line L370 (79.3694, -18.524) -> (79.1008, -18.6878)
  line L371 (79.1008, -18.6878) -> (78.8831, -18.9092)
  line L372 (78.8831, -18.9092) -> (71.0895, -29.3266)
  line L373 (71.0895, -29.3266) -> (71.0228, -29.4705)
  line L374 (71.0228, -29.4705) -> (71.047, -29.6043)
  line L375 (71.047, -29.6043) -> (71.1437, -29.7012)
  line L376 (71.1437, -29.7012) -> (71.2948, -29.7347)
  line L377 (71.2948, -29.7347) -> (74.0884, -29.7373)
  line L378 (74.0884, -29.7373) -> (74.3255, -29.7016)
  line L379 (74.3255, -29.7016) -> (74.5444, -29.608)
  line L380 (74.5444, -29.608) -> (74.8822, -29.3266)
  line L381 (74.8822, -29.3266) -> (75.5936, -28.398)
  line L382 (75.5936, -28.398) -> (75.7965, -28.2039)
  line L383 (75.7965, -28.2039) -> (76.0498, -28.1516)
  line L384 (76.0498, -28.1516) -> (80.2805, -28.1593)
  line L385 (80.2805, -28.1593) -> (80.4652, -28.2538)
  line L386 (80.4652, -28.2538) -> (80.5099, -28.4103)
  line L387 (80.5099, -28.4103) -> (80.4944, -29.3176)
  line L388 (80.4944, -29.3176) -> (80.593, -29.5984)
  line L389 (80.593, -29.5984) -> (80.7163, -29.6957)
  line L390 (80.7163, -29.6957) -> (80.8837, -29.7347)
  line L391 (80.8837, -29.7347) -> (85.0165, -29.7347)
  line L392 (85.0165, -29.7347) -> (85.344, -29.6297)
  line L393 (85.344, -29.6297) -> (85.4356, -29.5011)
  line L394 (85.4356, -29.5011) -> (85.4732, -29.324)
  line L395 (85.4732, -29.324) -> (85.7224, -18.9009)
  line L396 (85.7224, -18.9009) -> (85.6986, -18.6832)
  line L397 (85.6986, -18.6832) -> (85.609, -18.522)
  line L398 (85.609, -18.522) -> (85.4468, -18.4219)
  line L399 (85.4468, -18.4219) -> (85.205, -18.3876)
  line L400 (98.5111, -26.4511) -> (94.9793, -26.4511)
  line L401 (94.9793, -26.4511) -> (94.4769, -26.5252)
  line L402 (94.4769, -26.5252) -> (94.1611, -26.7098)
  line L403 (94.1611, -26.7098) -> (93.9668, -26.9484)
  line L404 (93.9668, -26.9484) -> (93.8289, -27.1846)
  line L405 (93.8289, -27.1846) -> (93.6419, -27.4267)
  line L406 (93.6419, -27.4267) -> (93.4298, -27.5918)
  line L407 (93.4298, -27.5918) -> (93.1968, -27.6873)
  line L408 (93.1968, -27.6873) -> (92.9472, -27.7204)
  line L409 (92.9472, -27.7204) -> (92.5949, -27.7217)
  line L410 (92.5949, -27.7217) -> (92.2401, -27.6644)
  line L411 (92.2401, -27.6644) -> (92.055, -27.4875)
  line L412 (92.055, -27.4875) -> (92.0343, -27.1893)
  line L413 (92.0343, -27.1893) -> (92.1728, -26.7681)
  line L414 (92.1728, -26.7681) -> (94.7861, -21.1475)
  line L415 (94.7861, -21.1475) -> (94.9834, -20.8118)
  line L416 (94.9834, -20.8118) -> (95.2297, -20.5618)
  line L417 (95.2297, -20.5618) -> (95.5295, -20.4088)
  line L418 (95.5295, -20.4088) -> (95.8874, -20.364)
  line L419 (95.8874, -20.364) -> (96.5954, -20.3736)
  line L420 (96.5954, -20.3736) -> (96.8411, -20.4356)
  line L421 (96.8411, -20.4356) -> (97.0266, -20.5971)
  line L422 (97.0266, -20.5971) -> (97.1228, -20.8208)
  line L423 (97.1228, -20.8208) -> (97.1003, -21.0699)
  line L424 (97.1003, -21.0699) -> (97.0339, -21.3932)
  line L425 (97.0339, -21.3932) -> (97.0864, -21.6604)
  line L426 (97.0864, -21.6604) -> (97.2596, -21.8421)
  line L427 (97.2596, -21.8421) -> (97.5556, -21.9092)
  line L428 (97.5556, -21.9092) -> (100.7243, -21.9092)
  line L429 (100.7243, -21.9092) -> (101.0334, -21.8697)
  line L430 (101.0334, -21.8697) -> (101.3049, -21.7582)
  line L431 (101.3049, -21.7582) -> (101.5373, -21.585)
  line L432 (101.5373, -21.585) -> (101.7294, -21.3602)
  line L433 (101.7294, -21.3602) -> (101.9866, -20.7976)
  line L434 (101.9866, -20.7976) -> (102.0654, -20.1525)
  line L435 (102.0654, -20.1525) -> (101.9545, -19.5075)
  line L436 (101.9545, -19.5075) -> (101.6427, -18.9448)
  line L437 (101.6427, -18.9448) -> (101.408, -18.7201)
  line L438 (101.408, -18.7201) -> (101.1188, -18.5468)
  line L439 (101.1188, -18.5468) -> (100.7738, -18.4353)
  line L440 (100.7738, -18.4353) -> (100.3716, -18.3959)
  line L441 (100.3716, -18.3959) -> (93.1153, -18.3959)
  line L442 (93.1153, -18.3959) -> (92.6089, -18.4355)
  line L443 (92.6089, -18.4355) -> (92.1317, -18.5515)
  line L444 (92.1317, -18.5515) -> (91.686, -18.7396)
  line L445 (91.686, -18.7396) -> (91.2742, -18.9954)
  line L446 (91.2742, -18.9954) -> (90.8984, -19.3145)
  line L447 (90.8984, -19.3145) -> (90.5611, -19.6926)
  line L448 (90.5611, -19.6926) -> (90.0109, -20.6085)
  line L449 (90.0109, -20.6085) -> (86.8784, -27.3675)
  line L450 (86.8784, -27.3675) -> (86.6944, -27.8909)
  line L451 (86.6944, -27.8909) -> (86.6443, -28.3574)
  line L452 (86.6443, -28.3574) -> (86.7084, -28.7629)
  line L453 (86.7084, -28.7629) -> (86.8673, -29.1036)
  line L454 (86.8673, -29.1036) -> (87.1013, -29.3755)
  line L455 (87.1013, -29.3755) -> (87.3908, -29.5746)
  line L456 (87.3908, -29.5746) -> (87.7164, -29.6969)
  line L457 (87.7164, -29.6969) -> (88.0585, -29.7386)
  line L458 (88.0585, -29.7386) -> (95.8417, -29.7386)
  line L459 (95.8417, -29.7386) -> (96.3703, -29.7017)
  line L460 (96.3703, -29.7017) -> (96.8543, -29.5973)
  line L461 (96.8543, -29.5973) -> (97.2929, -29.4352)
  line L462 (97.2929, -29.4352) -> (97.6854, -29.2249)
  line L463 (97.6854, -29.2249) -> (98.3287, -28.6984)
  line L464 (98.3287, -28.6984) -> (98.7781, -28.0948)
  line L465 (98.7781, -28.0948) -> (99.0272, -27.4913)
  line L466 (99.0272, -27.4913) -> (99.0699, -26.9648)
  line L467 (99.0699, -26.9648) -> (99.0119, -26.7545)
  line L468 (99.0119, -26.7545) -> (98.9, -26.5924)
  line L469 (98.9, -26.5924) -> (98.7333, -26.488)
  line L470 (98.7333, -26.488) -> (98.5111, -26.4511)
  line L471 (39.9499, -26.4511) -> (36.418, -26.4511)
  line L472 (36.418, -26.4511) -> (35.916, -26.5252)
  line L473 (35.916, -26.5252) -> (35.6, -26.7098)
  line L474 (35.6, -26.7098) -> (35.4052, -26.9484)
  line L475 (35.4052, -26.9484) -> (35.2667, -27.1846)
  line L476 (35.2667, -27.1846) -> (35.0809, -27.4267)
  line L477 (35.0809, -27.4267) -> (34.8691, -27.5918)
  line L478 (34.8691, -27.5918) -> (34.6361, -27.6873)
  line L479 (34.6361, -27.6873) -> (34.3864, -27.7204)
  line L480 (34.3864, -27.7204) -> (34.0353, -27.7217)
  line L481 (34.0353, -27.7217) -> (33.6798, -27.6644)
  line L482 (33.6798, -27.6644) -> (33.4943, -27.4875)
  line L483 (33.4943, -27.4875) -> (33.4738, -27.1893)
  line L484 (33.4738, -27.1893) -> (33.6131, -26.7681)
  line L485 (33.6131, -26.7681) -> (36.2255, -21.1475)
  line L486 (36.2255, -21.1475) -> (36.4235, -20.8118)
  line L487 (36.4235, -20.8118) -> (36.6696, -20.5618)
  line L488 (36.6696, -20.5618) -> (36.9687, -20.4088)
  line L489 (36.9687, -20.4088) -> (37.326, -20.364)
  line L490 (37.326, -20.364) -> (38.0338, -20.3736)
  line L491 (38.0338, -20.3736) -> (38.2792, -20.4356)
  line L492 (38.2792, -20.4356) -> (38.4651, -20.5971)
  line L493 (38.4651, -20.5971) -> (38.5616, -20.8208)
  line L494 (38.5616, -20.8208) -> (38.5388, -21.0699)
  line L495 (38.5388, -21.0699) -> (38.4732, -21.3932)
  line L496 (38.4732, -21.3932) -> (38.526, -21.6604)
  line L497 (38.526, -21.6604) -> (38.6993, -21.8421)
  line L498 (38.6993, -21.8421) -> (38.995, -21.9092)
  line L499 (38.995, -21.9092) -> (42.1644, -21.9092)
  line L500 (42.1644, -21.9092) -> (42.4733, -21.8697)
  line L501 (42.4733, -21.8697) -> (42.7447, -21.7582)
  line L502 (42.7447, -21.7582) -> (42.977, -21.585)
  line L503 (42.977, -21.585) -> (43.169, -21.3602)
  line L504 (43.169, -21.3602) -> (43.426, -20.7976)
  line L505 (43.426, -20.7976) -> (43.5046, -20.1525)
  line L506 (43.5046, -20.1525) -> (43.3935, -19.5075)
  line L507 (43.3935, -19.5075) -> (43.0815, -18.9448)
  line L508 (43.0815, -18.9448) -> (42.8466, -18.7201)
  line L509 (42.8466, -18.7201) -> (42.5572, -18.5468)
  line L510 (42.5572, -18.5468) -> (42.212, -18.4353)
  line L511 (42.212, -18.4353) -> (41.8095, -18.3959)
  line L512 (41.8095, -18.3959) -> (34.5525, -18.3959)
  line L513 (34.5525, -18.3959) -> (34.047, -18.4355)
  line L514 (34.047, -18.4355) -> (33.5704, -18.5515)
  line L515 (33.5704, -18.5515) -> (33.1251, -18.7396)
  line L516 (33.1251, -18.7396) -> (32.7134, -18.9954)
  line L517 (32.7134, -18.9954) -> (32.3378, -19.3145)
  line L518 (32.3378, -19.3145) -> (32.0004, -19.6926)
  line L519 (32.0004, -19.6926) -> (31.4499, -20.6085)
  line L520 (31.4499, -20.6085) -> (28.3178, -27.3675)
  line L521 (28.3178, -27.3675) -> (28.1334, -27.8909)
  line L522 (28.1334, -27.8909) -> (28.083, -28.3574)
  line L523 (28.083, -28.3574) -> (28.1471, -28.7629)
  line L524 (28.1471, -28.7629) -> (28.3059, -29.1036)
  line L525 (28.3059, -29.1036) -> (28.5399, -29.3755)
  line L526 (28.5399, -29.3755) -> (28.8294, -29.5746)
  line L527 (28.8294, -29.5746) -> (29.1548, -29.6969)
  line L528 (29.1548, -29.6969) -> (29.4966, -29.7386)
  line L529 (29.4966, -29.7386) -> (37.2804, -29.7386)
  line L530 (37.2804, -29.7386) -> (37.809, -29.7017)
  line L531 (37.809, -29.7017) -> (38.2929, -29.5973)
  line L532 (38.2929, -29.5973) -> (38.7315, -29.4352)
  line L533 (38.7315, -29.4352) -> (39.1239, -29.2249)
  line L534 (39.1239, -29.2249) -> (39.7672, -28.6984)
  line L535 (39.7672, -28.6984) -> (40.2166, -28.0948)
  line L536 (40.2166, -28.0948) -> (40.4658, -27.4913)
  line L537 (40.4658, -27.4913) -> (40.5085, -26.9648)
  line L538 (40.5085, -26.9648) -> (40.4506, -26.7545)
  line L539 (40.4506, -26.7545) -> (40.3387, -26.5924)
  line L540 (40.3387, -26.5924) -> (40.172, -26.488)
  line L541 (40.172, -26.488) -> (39.9499, -26.4511)
  line L542 (117.0857, -18.9138) -> (117.1888, -18.6965)
  line L543 (117.1888, -18.6965) -> (117.1689, -18.5283)
  line L544 (117.1689, -18.5283) -> (117.0555, -18.4197)
  line L545 (117.0555, -18.4197) -> (116.8779, -18.3811)
  line L546 (116.8779, -18.3811) -> (114.0507, -18.3856)
  line L547 (114.0507, -18.3856) -> (113.5158, -18.4461)
  line L548 (113.5158, -18.4461) -> (113.2276, -18.5681)
  line L549 (113.2276, -18.5681) -> (112.9641, -18.7925)
  line L550 (112.9641, -18.7925) -> (110.9318, -21.1238)
  line L551 (110.9318, -21.1238) -> (109.2232, -23.0238)
  line L552 (109.2232, -23.0238) -> (109.042, -23.1665)
  line L553 (109.042, -23.1665) -> (108.8142, -23.2609)
  line L554 (108.8142, -23.2609) -> (108.2932, -23.3407)
  line L555 (108.2932, -23.3407) -> (107.5106, -23.3177)
  line L556 (107.5106, -23.3177) -> (107.7568, -22.7511)
  line L557 (107.7568, -22.7511) -> (109.541, -18.8906)
  line L558 (109.541, -18.8906) -> (109.5227, -18.5816)
  line L559 (109.5227, -18.5816) -> (109.4189, -18.4491)
  line L560 (109.4189, -18.4491) -> (109.2513, -18.3933)
  line L561 (109.2513, -18.3933) -> (105.5367, -18.3856)
  line L562 (105.5367, -18.3856) -> (105.3159, -18.423)
  line L563 (105.3159, -18.423) -> (105.1108, -18.5283)
  line L564 (105.1108, -18.5283) -> (104.7972, -18.9016)
  line L565 (104.7972, -18.9016) -> (100.0969, -29.0924)
  line L566 (100.0969, -29.0924) -> (100.0421, -29.3332)
  line L567 (100.0421, -29.3332) -> (100.0961, -29.544)
  line L568 (100.0961, -29.544) -> (100.2317, -29.6933)
  line L569 (100.2317, -29.6933) -> (100.4216, -29.7501)
  line L570 (100.4216, -29.7501) -> (103.9823, -29.7386)
  line L571 (103.9823, -29.7386) -> (104.3796, -29.635)
  line L572 (104.3796, -29.635) -> (104.6644, -29.3356)
  line L573 (104.6644, -29.3356) -> (106.3369, -25.7729)
  line L574 (106.3369, -25.7729) -> (106.4669, -25.5865)
  line L575 (106.4669, -25.5865) -> (106.5866, -25.5067)
  line L576 (106.5866, -25.5067) -> (106.7522, -25.4738)
  line L577 (106.7522, -25.4738) -> (107.8154, -25.4738)
  line L578 (107.8154, -25.4738) -> (108.0401, -25.5742)
  line L579 (108.0401, -25.5742) -> (108.1565, -25.8499)
  line L580 (108.1565, -25.8499) -> (109.0473, -29.0937)
  line L581 (109.0473, -29.0937) -> (109.2341, -29.5533)
  line L582 (109.2341, -29.5533) -> (109.3727, -29.6968)
  line L583 (109.3727, -29.6968) -> (109.5557, -29.7501)
  line L584 (109.5557, -29.7501) -> (113.2465, -29.7386)
  line L585 (113.2465, -29.7386) -> (113.4586, -29.6723)
  line L586 (113.4586, -29.6723) -> (113.6248, -29.5085)
  line L587 (113.6248, -29.5085) -> (113.7132, -29.2778)
  line L588 (113.7132, -29.2778) -> (113.6919, -29.0109)
  line L589 (113.6919, -29.0109) -> (112.489, -25.0522)
  line L590 (112.489, -25.0522) -> (112.3959, -24.5967)
  line L591 (112.3959, -24.5967) -> (112.3992, -24.2905)
  line L592 (112.3992, -24.2905) -> (112.504, -24.0377)
  line L593 (112.504, -24.0377) -> (115.3458, -20.8556)
  line L594 (115.3458, -20.8556) -> (117.0857, -18.9138)
  line L595 (58.914, -18.3933) -> (55.1498, -18.3844)
  line L596 (55.1498, -18.3844) -> (54.9294, -18.4215)
  line L597 (54.9294, -18.4215) -> (54.7242, -18.5263)
  line L598 (54.7242, -18.5263) -> (54.4112, -18.9003)
  line L599 (54.4112, -18.9003) -> (52.6076, -22.8397)
  line L600 (52.6076, -22.8397) -> (52.4241, -23.0469)
  line L601 (52.4241, -23.0469) -> (52.1423, -23.1445)
  line L602 (52.1423, -23.1445) -> (49.0637, -23.1445)
  line L603 (49.0637, -23.1445) -> (48.949, -23.1112)
  line L604 (48.949, -23.1112) -> (48.8663, -23.0226)
  line L605 (48.8663, -23.0226) -> (48.8325, -22.8951)
  line L606 (48.8325, -22.8951) -> (48.8645, -22.7453)
  line L607 (48.8645, -22.7453) -> (50.6462, -18.89)
  line L608 (50.6462, -18.89) -> (50.6287, -18.5791)
  line L609 (50.6287, -18.5791) -> (50.5255, -18.4467)
  line L610 (50.5255, -18.4467) -> (50.359, -18.3914)
  line L611 (50.359, -18.3914) -> (46.6448, -18.3844)
  line L612 (46.6448, -18.3844) -> (46.4247, -18.4215)
  line L613 (46.4247, -18.4215) -> (46.2195, -18.5263)
  line L614 (46.2195, -18.5263) -> (45.9054, -18.9003)
  line L615 (45.9054, -18.9003) -> (41.2095, -29.0815)
  line L616 (41.2095, -29.0815) -> (41.1548, -29.3223)
  line L617 (41.1548, -29.3223) -> (41.2085, -29.533)
  line L618 (41.2085, -29.533) -> (41.3439, -29.6824)
  line L619 (41.3439, -29.6824) -> (41.5342, -29.7392)
  line L620 (41.5342, -29.7392) -> (45.0926, -29.727)
  line L621 (43.7874, -29.7597) -> (45.4892, -29.6235)
  line L622 (45.4892, -29.6235) -> (45.7739, -29.3246)
  line L623 (45.7739, -29.3246) -> (47.5335, -25.5881)
  line L624 (47.5335, -25.5881) -> (47.7142, -25.4013)
  line L625 (47.7142, -25.4013) -> (48.0513, -25.2897)
  line L626 (48.0513, -25.2897) -> (51.0243, -25.2897)
  line L627 (51.0243, -25.2897) -> (51.2722, -25.3982)
  line L628 (51.2722, -25.3982) -> (51.32, -25.5143)
  line L629 (51.32, -25.5143) -> (51.2908, -25.665)
  line L630 (51.2908, -25.665) -> (49.714, -29.0815)
  line L631 (49.714, -29.0815) -> (49.6593, -29.3223)
  line L632 (49.6593, -29.3223) -> (49.7133, -29.533)
  line L633 (49.7133, -29.533) -> (49.8488, -29.6824)
  line L634 (49.8488, -29.6824) -> (50.0386, -29.7392)
  line L635 (50.0386, -29.7392) -> (53.7476, -29.727)
  line L636 (53.7476, -29.727) -> (54.1441, -29.6235)
  line L637 (54.1441, -29.6235) -> (54.428, -29.3246)
  line L638 (54.428, -29.3246) -> (59.2568, -18.9824)
  line L639 (59.2568, -18.9824) -> (59.2981, -18.7888)
  line L640 (59.2981, -18.7888) -> (59.2653, -18.5976)
  line L641 (59.2653, -18.5976) -> (59.1426, -18.4515)
  line L642 (59.1426, -18.4515) -> (58.914, -18.3933)
  line L643 (24.9277, -22.7562) -> (22.4128, -21.423)
  line L644 (22.4128, -21.423) -> (19.1043, -19.6196)
  line L645 (19.1043, -19.6196) -> (18.7872, -19.345)
  line L646 (18.7872, -19.345) -> (18.6199, -19.0094)
  line L647 (18.6199, -19.0094) -> (18.5865, -18.6429)
  line L648 (18.5865, -18.6429) -> (18.6712, -18.2757)
  line L649 (18.6712, -18.2757) -> (18.8579, -17.9377)
  line L650 (18.8579, -17.9377) -> (19.131, -17.659)
  line L651 (19.131, -17.659) -> (19.4745, -17.4698)
  line L652 (19.4745, -17.4698) -> (19.8724, -17.4)
  line L653 (19.8724, -17.4) -> (22.7446, -17.4)
  line L654 (22.7446, -17.4) -> (23.003, -17.443)
  line L655 (23.003, -17.443) -> (23.1756, -17.5725)
  line L656 (23.1756, -17.5725) -> (23.2451, -17.789)
  line L657 (23.2451, -17.789) -> (23.1945, -18.093)
  line L658 (23.1945, -18.093) -> (23.1482, -18.4518)
  line L659 (23.1482, -18.4518) -> (23.2643, -18.7075)
  line L660 (23.2643, -18.7075) -> (23.5148, -18.8594)
  line L661 (23.5148, -18.8594) -> (23.8721, -18.9067)
  line L662 (23.8721, -18.9067) -> (28.7022, -18.8829)
  line L663 (28.7022, -18.8829) -> (29.0413, -18.8386)
  line L664 (29.0413, -18.8386) -> (29.3187, -18.723)
  line L665 (29.3187, -18.723) -> (29.5351, -18.5464)
  line L666 (29.5351, -18.5464) -> (29.691, -18.319)
  line L667 (29.691, -18.319) -> (29.7873, -18.051)
  line L668 (29.7873, -18.051) -> (29.8244, -17.7526)
  line L669 (29.8244, -17.7526) -> (29.7242, -17.1057)
  line L670 (29.7242, -17.1057) -> (29.3956, -16.4602)
  line L671 (29.3956, -16.4602) -> (28.844, -15.8978)
  line L672 (28.844, -15.8978) -> (28.4862, -15.6734)
  line L673 (28.4862, -15.6734) -> (28.0746, -15.5004)
  line L674 (28.0746, -15.5004) -> (27.6099, -15.3891)
  line L675 (27.6099, -15.3891) -> (27.0928, -15.3497)
  line L676 (27.0928, -15.3497) -> (17.0907, -15.3497)
  line L677 (17.0907, -15.3497) -> (16.475, -15.3795)
  line L678 (16.475, -15.3795) -> (15.8803, -15.4742)
  line L679 (15.8803, -15.4742) -> (15.3121, -15.6416)
  line L680 (15.3121, -15.6416) -> (14.7756, -15.8897)
  line L681 (14.7756, -15.8897) -> (14.2762, -16.2264)
  line L682 (14.2762, -16.2264) -> (13.8193, -16.6595)